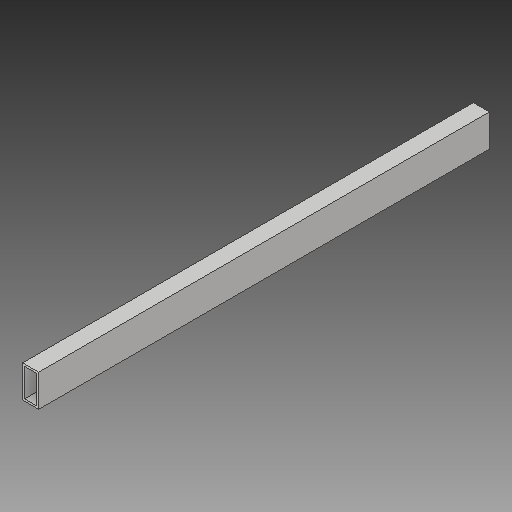
# Autodesk Inventor part: 23 Alum Tube
Saved by Autodesk Inventor 2018.2 (Build 222227000, 227)
## iProperties
Created: 2018-01-13
Part Number: 23 Alum Tube
Material: Generic
Document SubType Name: Modeling
Designer: Orangeracer
Density: 1 g/cm^3
Appearance: Default
Mass: 315.451 g
Surface Area: 1995.96 cm^2
Volume: 315.451 cm^3
Author: Orangeracer
Autodesk Inventor part; units mm, degrees
ref_plane "YZ Plane" through (0, 0, 0) normal (1, 0, 0) x (0, 1, 0)
ref_plane "XZ Plane" through (0, 0, 0) normal (0, 1, 0) x (-1, 0, 0)
ref_plane "XY Plane" through (0, 0, 0) normal (0, 0, 1) x (1, 0, 0)
sketch "Sketch1" plane through (0, 0, 0) normal (0, 0, 1) x (1, 0, 0)
  line L0 (0, 0) -> (-25.4, 0)
  line L1 (-25.4, 0) -> (-25.4, 50.8)
  line L2 (-25.4, 50.8) -> (0, 50.8)
  line L3 (0, 50.8) -> (0, 0)
  line L4 (-22.225, 3.175) -> (-3.175, 3.175)
  line L5 (-3.175, 3.175) -> (-3.175, 47.625)
  line L6 (-3.175, 47.625) -> (-22.225, 47.625)
  line L7 (-22.225, 47.625) -> (-22.225, 3.175)
  dimension "d0" = 25.4
  dimension "d1" = 50.8
  dimension "d2" = 3.175
  constraints: 16 end point, 4 parallel, 2 perpendicular, 1 horizontal, 3 other
  measures "d0" distance of L1.end L2.end
  measures "d1" distance of L0.end L1.end
  measures "d2" distance between parallel lines of L0 L4
extrude "Extrusion1" add sketch "Sketch1" along normal blind 711.2
body "Solid1"
